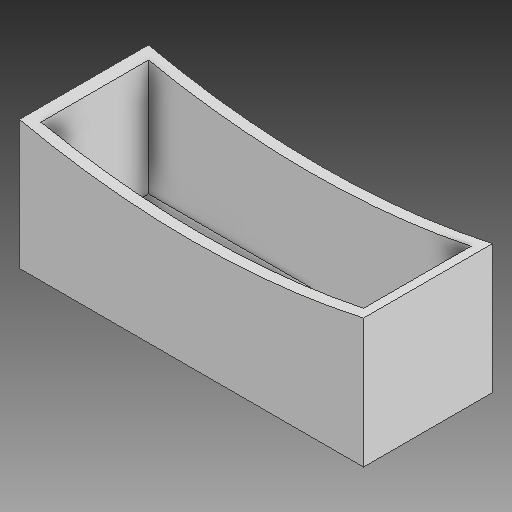
# Autodesk Inventor part: WasserAblauf1
Saved by Autodesk Inventor 2021 (Build 250183000, 183)
## iProperties
Created: 2022-02-02
Part Number: WasserAblauf1
Material: Generisch
Document SubType Name: Modeling
Designer: lukas
Density: 1 g/cm^3
Appearance: Vorgabe
Stock Number: Wasserablauf
Author: lukas
Autodesk Inventor part; units mm, degrees
ref_plane "YZ Plane" through (0, 0, 0) normal (1, 0, 0) x (0, 1, 0)
ref_plane "XZ Plane" through (0, 0, 0) normal (0, 1, 0) x (-1, 0, 0)
ref_plane "XY Plane" through (0, 0, 0) normal (0, 0, 1) x (1, 0, 0)
sketch "Skizze1" plane through (0, 0, 0) normal (0, 0, 1) x (1, 0, 0)
  line L0 (-259, 0) -> (259, 0) projected
  line L1 (0, -289.7487) -> (0, 264.1248) projected
  circle A0 centre (0, 0) radius 185
  line L2 (-40, -180.6239) -> (40, -180.6239)
  line L3 (-40, -180.6239) -> (-40, -210.6239)
  line L4 (-40, -210.6239) -> (40, -210.6239)
  line L5 (40, -210.6239) -> (40, -180.6239)
  point P0 (0, -180.6239)
  dimension "d0" = 370
  dimension "d1" = 80
  dimension "d2" = 40
  dimension "d3" = 0
  dimension "d4" = 30
  constraints: 8 end point, 3 coincident, 2 perpendicular, 1 horizontal, 1 midpoint, 1 point on line, 1 vertical, 3 other
  measures "d1" distance of L2.start L2.end
  measures "d2" distance of L2.end point (0, -180.624)
  measures "d3" distance of L2.start L3.start
  measures "d4" distance of L3.start L3.end
extrude "Extrusion1" add sketch "Skizze1" along normal blind 30 contours A0 L1 L4 L3 | A0 L5 L4 L1
sketch "Skizze2" plane through (-40, -210.6239, 0) normal (0, -1, 0) x (1, 0, 0)
  point P0 (40, 0)
sketch "Skizze3" plane through (-40, -210.6239, 0) normal (0, -1, 0) x (1, 0, 0)
  line L0 (2.5, 2.5) -> (77.5, 2.5)
  line L1 (77.5, 2.5) -> (77.5, 27.5)
  line L2 (77.5, 27.5) -> (2.5, 27.5)
  line L3 (2.5, 27.5) -> (2.5, 2.5)
  line L4 (0, 0) -> (0, 30) projected
  line L5 (0, 0) -> (80, 0) projected
  line L6 (0, 30) -> (80, 30) projected
  line L7 (80, 0) -> (80, 30) projected
  point P0 (40, 0)
  dimension "d7" = 2.5
  dimension "d8" = 2.5
  dimension "d9" = 2.5
  dimension "d10" = 2.5
  constraints: 8 end point, 2 parallel, 1 horizontal, 1 perpendicular
  measures "d7" distance between parallel lines of L4 L3
  measures "d8" distance between parallel lines of L5 L0
  measures "d9" distance between parallel lines of L6 L2
  measures "d10" distance between parallel lines of L7 L1
extrude "Extrusion2" cut sketch "Skizze3" against normal blind 30 contours L3 L2 L1 L0
sketch "Skizze4" plane through (-40, -210.6239, 0) normal (0, -1, 0) x (1, 0, 0)
  line L0 (2.5, 27.5) -> (2.5, 2.5) projected
  line L1 (77.5, 27.5) -> (77.5, 2.5) projected
  line L2 (2.5, 2.5) -> (77.5, 2.5)
  line L3 (77.5, 2.5) -> (77.5, 27.5)
  line L4 (77.5, 27.5) -> (2.5, 27.5)
  line L5 (2.5, 27.5) -> (2.5, 2.5)
  point P0 (40, 0)
  constraints: 8 end point, 2 parallel, 1 horizontal, 1 perpendicular
extrude "Extrusion3" add sketch "Skizze4" against normal blind 2.5
sketch "Skizze5" plane through (-40, -210.6239, 0) normal (0, -1, 0) x (1, 0, 0)
  line L0 (0, 0) -> (0, 30) projected
  point P0 (40, 0)
  point P1 (40, 15)
  dimension "d15" = 40
  dimension "d16" = 15
  measures "d15" distance from line of point (40, 15) L0
  measures "d16" distance of point (40, 0) point (40, 15)
hole "Bohrung1" at (0, -210.6239, 15) direction (0, 1, 0) diameter 9.3762 end through all thread size "M11x1.5" class "6H" standard "ISO Metric profile"
